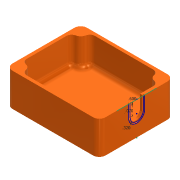
# Autodesk Inventor part: Machined Base
Saved by Autodesk Inventor 2020.1 (Build 241239000, 239)
## iProperties
Created: 2019-10-07
Part Number: Machined Base
Material: Steel, Mild
Document SubType Name: Modeling
Designer: thom_tremblay
Density: 7.85 g/cm^3
Appearance: Smooth - Light Orange
Author: thom_tremblay
Autodesk Inventor part; units mm, degrees
ref_plane "YZ Plane" through (0, 0, 0) normal (1, 0, 0) x (0, 1, 0)
ref_plane "XZ Plane" through (0, 0, 0) normal (0, 1, 0) x (-1, 0, 0)
ref_plane "XY Plane" through (0, 0, 0) normal (0, 0, 1) x (1, 0, 0)
sketch "Sketch1" plane through (0, 0, 0) normal (0, 1, 0) x (-1, 0, 0)
  line L0 (57.15, 45.72) -> (-57.15, 45.72)
  line L1 (-57.15, 45.72) -> (-57.15, -45.72)
  line L2 (-57.15, -45.72) -> (57.15, -45.72)
  line L3 (57.15, -45.72) -> (57.15, 45.72)
  point P0 (0, 0)
  point P1 (-57.15, 0)
  point P2 (0, -45.72)
  dimension "d0" = 114.3
  dimension "d1" = 91.44
  constraints: 8 end point, 2 midpoint, 2 parallel, 1 horizontal, 1 horizontal alignment, 1 perpendicular, 1 vertical alignment
  measures "d0" distance of L2.end L1.end
  measures "d1" distance of L1.end L0.end
extrude "Extrusion1" add sketch "Sketch1" along normal blind 40.64
fillet "Fillet1" radius 7.62 4 edges at (-57.15, 20.32, 45.72) (57.15, 20.32, 45.72) (-57.15, 20.32, -45.72) (57.15, 20.32, -45.72)
sketch "Sketch2" plane through (0, 40.64, 0) normal (0, 1, 0) x (1, 0, 0)
  arc A0 (-57.15, -38.1) -> (-49.53, -45.72) centre (-49.53, -38.1) ccw projected
  line L0 (-57.15, 38.1) -> (-57.15, -38.1) projected
  circle A1 centre (-49.53, -38.1) radius 7.62
  arc A2 (-49.53, 45.72) -> (-57.15, 38.1) centre (-49.53, 38.1) ccw projected
  circle A3 centre (-49.53, 38.1) radius 7.62
  arc A4 (57.15, 38.1) -> (49.53, 45.72) centre (49.53, 38.1) ccw projected
  line L1 (49.53, 45.72) -> (-49.53, 45.72) projected
  circle A5 centre (49.53, 38.1) radius 7.62
  arc A6 (49.53, -45.72) -> (57.15, -38.1) centre (49.53, -38.1) ccw projected
  circle A7 centre (49.53, -38.1) radius 7.62
  line L2 (-53.34, -41.91) -> (53.34, -41.91)
  line L3 (53.34, -41.91) -> (53.34, 41.91)
  line L4 (53.34, 41.91) -> (-53.34, 41.91)
  line L5 (-53.34, 41.91) -> (-53.34, -41.91)
  point P0 (0, 0)
  point P1 (-53.34, 0)
  point P2 (0, 41.91)
  point P3 (-53.34, 31.5009)
  point P4 (-53.34, -31.5009)
  point P5 (-42.9309, -41.91)
  point P6 (42.9309, -41.91)
  point P7 (53.34, -31.5009)
  point P8 (53.34, 31.5009)
  point P9 (42.9309, 41.91)
  point P10 (-42.9309, 41.91)
  dimension "d5" = 3.81
  dimension "d6" = 3.81
  constraints: 8 end point, 4 coincident, 2 midpoint, 2 parallel, 1 horizontal, 1 horizontal alignment, 1 perpendicular, 1 vertical alignment, 12 other
  measures "d5" distance between parallel lines of L0 L5
  measures "d6" distance between parallel lines of L1 L4
extrude "Extrusion2" cut sketch "Sketch2" against normal blind 34.29 contours L5 A3 L4 A5 L3 A7 L2 A1
fillet "Fillet2" radius 6.35 16 edges at (-42.9309, 23.495, 41.91) (-53.34, 23.495, 31.5009) (0, 6.35, 41.91) (-53.34, 6.35, 0) (-53.34, 23.495, -31.5009) (-44.1418, 6.35, -32.7118) (-42.9309, 23.495, -41.91) (-44.1418, 6.35, 32.7118) (44.1418, 6.35, 32.7118) (42.9309, 23.495, 41.91) (53.34, 23.495, 31.5009) (53.34, 6.35, 0) (44.1418, 6.35, -32.7118) (53.34, 23.495, -31.5009) (42.9309, 23.495, -41.91) (0, 6.35, -41.91)
sketch "Sketch3" plane through (57.15, 0, 38.1) normal (1, 0, 0) x (0, 0, -1)
  line L0 (13.7372, 40.64) -> (62.4628, 40.64) projected
  line L1 (29.972, 40.64) -> (29.972, 25.4)
  arc A0 (29.972, 25.4) -> (46.228, 25.4) centre (38.1, 25.4) ccw
  line L2 (46.228, 25.4) -> (46.228, 40.64)
  line L3 (28.194, 40.64) -> (28.194, 25.4)
  arc A1 (28.194, 25.4) -> (48.006, 25.4) centre (38.1, 25.4) ccw
  line L4 (48.006, 25.4) -> (48.006, 40.64)
  point P0 (38.1, 0)
  point P1 (38.1, 40.64)
  point P2 (28.194, 40.64)
  dimension "d10" = 15.24
  dimension "d11" = 8.128
  dimension "d12" = 1.778
  constraints: 8 end point, 4 point on circle, 2 centre point, 2 parallel, 2 point on line, 2 tangent, 1 midpoint, 1 vertical, 1 vertical alignment, 2 other
  measures "d10" distance of L1.start L1.end
  measures "d11" radius of A0
  measures "d12" distance between parallel lines of L1 L3
extrude "Extrusion3" cut sketch "Sketch3" against normal up to surface (3.81 mm away) contours L0 L2 A0 L1
extrude "Extrusion4" cut sketch "Sketch3" against normal blind 1.27 contours L0 L1 A0 L2 L4 A1 L3
equation "\"d6\" = d5"
body "Solid1"
